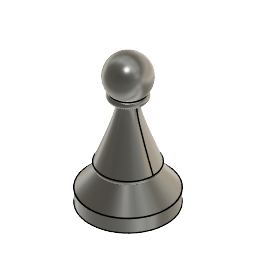
Pion (Autodesk Fusion 360 design; units mm, degrees)
part number: 2026-03-27-14-13-04-446
Autodesk Fusion 360 part; units mm, degrees
note: some values were not read from the file. Set by a fixed rule: which sketch regions a step uses.
sketch "Pion" plane through (0, 0, 0) normal (0, 1, 0) x (1, 0, 0)
  line L0 (0, 0) -> (12, 0)
  line L1 (12, 0) -> (12, -4) construction
  line L2 (0, 0) -> (0, -40) construction
  line L3 (6, 0) -> (6, -9.5696) construction
  line L4 (0, -30) -> (0, -28) construction
  line L5 (0, -30) -> (4, -30)
  line L6 (0, -28) -> (4, -28)
  arc A0 (4, -30) -> (5, -29) centre (4, -29) ccw
  arc A1 (5, -29) -> (4, -28) centre (4, -29) ccw
  line L7 (12, -4) -> (12, 0)
  line L8 (0, -40) -> (0, 0)
  line L9 (12, -4) -> (0, -4) construction
  line L10 (0, -9.6135) -> (6.9254, -9.6135)
  spline S0 degree 5 poles (7.8558, -10.9801) (7.5549, -11.7439) (6.8618, -13.5183) (5.8277, -16.2235) (4.5513, -19.7052) (3.268, -23.5962) (2.6775, -26.112) (2.6509, -27.3491) (2.8478, -27.8389) (3, -28) knots 0.052342 0.052342 0.052342 0.052342 0.052342 0.052342 0.2 0.4 0.6 0.8 1 1 1 1 1 1
  line L11 (2.6823, -27.6637) -> (3.3177, -28.3363)
  arc A2 (7.8558, -10.9801) -> (6.9254, -9.6135) centre (6.9254, -10.6135) ccw
  spline S1 degree 5 poles (6.9254, -9.6135) (7.1769, -9.3353) (7.6663, -8.794) (8.3596, -8.027) (9.2012, -7.0961) (10.1055, -6.0957) (10.8484, -5.274) (11.4156, -4.6465) (11.7977, -4.2238) (11.9996, -4.0005) (12.0478, -3.9472) (12.0208, -3.977) (12.0038, -3.9958) (12, -4) (12, -4) knots 0 0 0 0 0 0 0.1 0.2 0.3 0.4 0.5 0.6 0.7 0.8 0.9 1 1 1 1 1 1
  line L12 (12.2553, -4.7429) -> (11.7447, -3.257)
  arc A3 (0, -39.9814) -> (4.3789, -29.9254) centre (0, -34) ccw
  dimension "d1" = 12
  dimension "d2" = 4
  dimension "d3" = 40
  dimension "d5" = 2
  dimension "d6" = 1
  dimension "d7" = 1
  constraint coincident L0.start L2.start
  constraint horizontal L0
  constraint perpendicular L0 L1
  constraint perpendicular L0 L2
  constraint midpoint L0 L3.start
  constraint perpendicular L0 L3
  constraint coincident L2 L4.start
  constraint parallel L2 L4
  constraint perpendicular L4 L5
  constraint perpendicular L4 L6
  constraint tangent L5 A0
  constraint tangent L6 A1
  constraint equal A0 A1
  constraint coincident A0.end A1.start
  constraint coincident L1 L7.start
  constraint coincident L2 L9.end
  constraint perpendicular L2 L9
  constraint coincident L8 L10.start
  constraint perpendicular L3 L10
  constraint coincident L6 S0.end
  constraint midpoint S0.end L11
  constraint tangent L10 A2
  constraint tangent S0 A2
  constraint midpoint L1.end L12
  constraint coincident L2 A3.centre
  constraint coincident L2 A3.start
  constraint coincident A0 A3.end
  measures "d1" distance of L0.start L0.end
  measures "d2" distance of L0.end L1.end
  measures "d3" distance of L0.start L2.end
  measures "d5" distance of L4.start L4.end
  measures "d6" radius of A0
  measures "d7" radius of A2
revolve "Revolve1" add sketch "Pion" angle 360 about axis through (0, 0, 40) along (0, 0, -1)
named bodies: "Pion"
